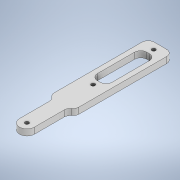
# Autodesk Inventor part: SideSensor
Saved by Autodesk Inventor 2022 (Build 260153000, 153)
## iProperties
Created: 2021-10-25
Part Number: SideSensor
Material: 一般
Document SubType Name: Modeling
Designer: shiok
Density: 1 g/cm^3
Appearance: 既定
Author: shiok
Autodesk Inventor part; units mm, degrees
ref_plane "YZ Plane" through (0, 0, 0) normal (1, 0, 0) x (0, 1, 0)
ref_plane "XZ Plane" through (0, 0, 0) normal (0, 1, 0) x (-1, 0, 0)
ref_plane "XY Plane" through (0, 0, 0) normal (0, 0, 1) x (1, 0, 0)
sketch "スケッチ1" plane through (0, 0, 0) normal (0, 1, 0) x (-1, 0, 0)
  line L0 (3, -32.5) -> (-3, -32.5)
  line L1 (-3, -32.5) -> (-3, -89.5)
  line L2 (3, -89.5) -> (3, -32.5)
  line L3 (-3, -89.5) -> (0, -89.5)
  line L4 (0, -89.5) -> (3, -89.5)
  point P0 (0, 0)
  point P1 (0, -35)
  point P2 (0, -40)
  point P3 (0, -50)
  dimension "d1" = 32.5
  dimension "d2" = 2.5
  dimension "d3" = 5
  dimension "d4" = 10
  dimension "d5" = 6
  dimension "d6" = 89.5
  constraints: 10 end point, 4 vertical alignment, 2 collinear, 2 horizontal, 1 parallel, 1 perpendicular
  measures "d1" distance from line of L0 point (0, 0)
  measures "d2" distance from line of L0 point (0, -35)
  measures "d3" distance of point (0, -40) point (0, -35)
  measures "d4" distance of point (0, -50) point (0, -40)
  measures "d5" distance of L0.start L0.end
  measures "d6" distance from line of point (0, 0) L4
extrude "押し出し1" add sketch "スケッチ1" along normal blind 2.5
sketch "スケッチ2" plane through (0, 2.5, 0) normal (0, 1, 0) x (1, 0, 0)
  line L0 (-3, 32.5) -> (3, 32.5) projected
  line L1 (0, 32.5) -> (0, 35) construction
  point P0 (0, 0)
  point P1 (0, 40)
  point P2 (0, 50)
  dimension "d9" = 2.5
  dimension "d10" = 5
  dimension "d11" = 10
  constraints: 2 end point, 2 vertical alignment, 1 midpoint, 1 vertical
  measures "d9" distance from line of L0 L1.end
  measures "d10" distance of point (0, 40) L1.end
  measures "d11" distance of point (0, 50) point (0, 40)
hole "穴1" at (0, 2.5, -50) at (0, 2.5, -40) at (0, 2.5, -35) direction (0, -1, 0) diameter 1.567 depth 2.5 tip angle 118 thread size "M2x0.4" class "6H" standard "ISO Metric profile"
sketch "スケッチ3" plane through (0, 2.5, 0) normal (0, 1, 0) x (1, 0, 0)
  line L0 (-5, 50) -> (-5, 89.5)
  line L1 (-5, 89.5) -> (5, 89.5)
  line L2 (5, 89.5) -> (5, 50)
  circle A0 centre (0, 50) radius 0.7835 projected
  line L3 (3, 89.5) -> (-3, 89.5) projected
  line L4 (5, 50) -> (0, 50)
  line L5 (0, 50) -> (-5, 50)
  point P0 (0, 0)
  point P1 (0.5, 89.5)
  point P2 (-0.5, 89.5)
  point P3 (-0.7835, 50)
  point P4 (0.7835, 50)
  dimension "d22" = 10
  constraints: 10 end point, 2 collinear, 2 equal length, 1 horizontal, 1 vertical
  measures "d22" distance between parallel lines of L2 L0
extrude "押し出し2" add sketch "スケッチ3" against normal up to surface (2.5 mm away) contours L0 L1 L2 L4 A0 L5
fillet "フィレット3" radius 2.5 6 edges at (5, 1.25, -50) (3, 1.25, -50) (-5, 1.25, -50) (-3, 1.25, -50) (5, 1.25, -89.5) (-5, 1.25, -89.5)
sketch "スケッチ4" plane through (0, 0, 0) normal (0, -1, 0) x (1, 0, 0)
  line L0 (-2.5, -89.5) -> (2.5, -89.5) projected
  line L1 (2.5, -89.5) -> (-2.5, -89.5) construction
  line L2 (0, -89.5) -> (0, -86.75) construction
  line L3 (0, -86.75) -> (0, -62.25) construction
  circle A0 centre (0, -50) radius 0.7835 projected
  point P0 (0, 0)
  point P1 (0, -74.5)
  dimension "d36" = 12.25
  dimension "d42" = 24.5
  constraints: 4 end point, 2 coincident, 2 midpoint, 1 point on line, 1 vertical
  measures "d36" distance of L3.end A0.centre
  measures "d42" distance of point (0, -86.75) point (0, -62.25)
hole "穴2" at (0, 0, -86.75) at (0, 0, -62.25) direction (0, 1, 0) diameter 1.567 depth 2.5 tip angle 118 thread size "M2x0.4" class "6H" standard "ISO Metric profile"
sketch "スケッチ5" plane through (0, 0, 0) normal (0, -1, 0) x (1, 0, 0)
  line L0 (-2.5, -89.5) -> (2.5, -89.5) projected
  line L1 (2.5, -89.5) -> (-2.5, -89.5) construction
  line L2 (0.5, -64.5) -> (-0.5, -64.5)
  line L3 (-3, -67) -> (-3, -82)
  line L4 (-0.5, -84.5) -> (0.5, -84.5)
  line L5 (3, -82) -> (3, -67)
  line L6 (3, -64.5) -> (-3, -84.5) construction
  line L7 (3, -84.5) -> (-3, -64.5) construction
  circle A0 centre (0, -62.25) radius 0.7835 construction
  circle A1 centre (0, -86.75) radius 0.7835 construction
  line L8 (0, -62.25) -> (0, -86.75) construction
  arc A2 (3, -67) -> (0.5, -64.5) centre (0.5, -67) ccw
  arc A3 (0.5, -84.5) -> (3, -82) centre (0.5, -82) ccw
  arc A4 (-3, -82) -> (-0.5, -84.5) centre (-0.5, -82) ccw
  arc A5 (-0.5, -64.5) -> (-3, -67) centre (-0.5, -67) ccw
  point P0 (0, 0)
  point P1 (0, -74.5)
  dimension "d37" = 20
  dimension "d38" = 6
  dimension "d39" = 2.5
  constraints: 14 end point, 8 point on circle, 8 point on line, 8 tangent, 4 centre point, 3 equal radius, 3 midpoint, 2 parallel, 1 horizontal, 1 perpendicular, 1 vertical
  measures "d37" distance of L7.end L6.end
  measures "d38" distance of L6.end L7.start
  measures "d39" radius of A2
extrude "押し出し3" cut sketch "スケッチ5" against normal up to surface (2.5 mm away)
sketch "スケッチ6" plane through (0, 2.5, 0) normal (0, 1, 0) x (1, 0, 0)
  circle A0 centre (0, 40) radius 0.7835 projected
  circle A1 centre (0, 35) radius 0.7835 projected
  point P0 (0, 0)
extrude "押し出し4" add sketch "スケッチ6" against normal up to surface (2.5 mm away)
sketch "スケッチ7" plane through (0, 2.5, 0) normal (0, 1, 0) x (1, 0, 0)
  line L0 (-3, 32.5) -> (3, 32.5) projected
  point P0 (0, 0)
  point P1 (0, 35.5)
  point P2 (0.5, 32.5)
  dimension "d45" = 3
  measures "d45" distance from line of point (0, 35.5) L0
hole "穴3" at (0, 2.5, -35.5) direction (0, -1, 0) diameter 1.567 depth 6.3 thread size "M2x0.4" class "6H" standard "ISO Metric profile"
fillet "フィレット4" radius 3 2 edges at (3, 1.25, -32.5) (-3, 1.25, -32.5)
sketch "スケッチ8" plane through (0, 2.5, 0) normal (0, 1, 0) x (1, 0, 0)
  circle A0 centre (0, 50) radius 0.7835 projected
  point P0 (0, 0)
extrude "押し出し5" add sketch "スケッチ8" against normal up to surface (2.5 mm away)
equation "\"d17\" = d11"
